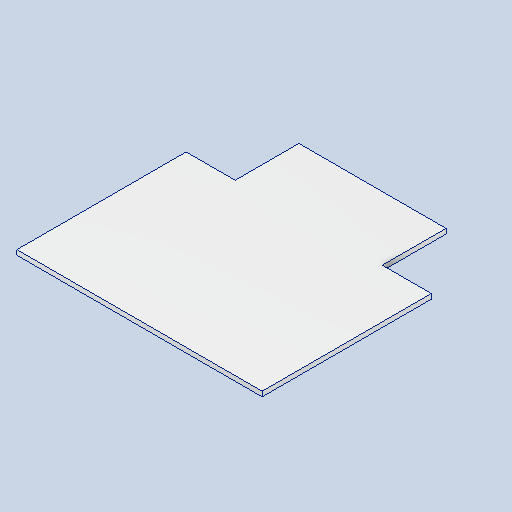
# Autodesk Inventor part: minisumopodsr
Saved by Autodesk Inventor 2022.3 (Build 263350000, 350)
## iProperties
Created: 2022-10-10
Part Number: minisumopodsr
Material: Aluminum 6061
Document SubType Name: Modeling
Designer: komputer
Density: 2.7 g/cm^3
Appearance: Aluminum - Flat
Author: komputer
Autodesk Inventor part; units mm, degrees
ref_plane "YZ Plane" through (0, 0, 0) normal (1, 0, 0) x (0, 1, 0)
ref_plane "XZ Plane" through (0, 0, 0) normal (0, 1, 0) x (-1, 0, 0)
ref_plane "XY Plane" through (0, 0, 0) normal (0, 0, 1) x (1, 0, 0)
sketch "Sketch1" plane through (0, 0, 0) normal (0, 1, 0) x (-1, 0, 0)
  line L0 (-95.7688, 101.9192) -> (4.2312, 101.9192)
  line L1 (4.2312, 101.9192) -> (4.2312, 1.9192)
  line L2 (4.2312, 1.9192) -> (-95.7688, 1.9192)
  line L3 (-95.7688, 1.9192) -> (-95.7688, 101.9192)
  line L4 (-95.7688, 1.9192) -> (4.2312, 1.9192)
  line L5 (4.2312, 1.9192) -> (4.2312, 6.9192)
  line L6 (4.2312, 6.9192) -> (-95.7688, 6.9192)
  line L7 (-95.7688, 6.9192) -> (-95.7688, 1.9192)
  line L8 (4.2312, 1.9192) -> (-15.7688, 1.9192)
  line L9 (-15.7688, 1.9192) -> (-15.7688, 32.9192)
  line L10 (-15.7688, 32.9192) -> (4.2312, 32.9192)
  line L11 (4.2312, 32.9192) -> (4.2312, 1.9192)
  line L12 (-95.7688, 1.9192) -> (-75.7688, 1.9192)
  line L13 (-75.7688, 1.9192) -> (-75.7688, 32.9192)
  line L14 (-75.7688, 32.9192) -> (-95.7688, 32.9192)
  line L15 (-95.7688, 32.9192) -> (-95.7688, 1.9192)
  point P0 (0, 0)
  dimension "d0" = 100
  dimension "d1" = 100
  dimension "d2" = 5
  dimension "d3" = 20
  dimension "d4" = 31
  dimension "d5" = 20
  constraints: 32 end point, 8 parallel, 4 horizontal, 4 perpendicular, 2 point on line
  measures "d0" distance of L1.end L2.end
  measures "d1" distance of L0.end L1.end
  measures "d2" distance of L5.end L4.end
  measures "d3" distance of L9.end L10.end
  measures "d4" distance of L8.end L9.end
  measures "d5" distance of L14.end L13.end
extrude "Extrusion1" add sketch "Sketch1" along normal blind 2 contours L0 L1 L10 L9 L6 L13 L14 L3 | L6 L9 L2 L13
sketch "Sketch2" plane through (0, 2, 0) normal (0, 1, 0) x (1, 0, 0)
  line L0 (-4.2312, -82.6348) -> (-4.2312, -11.6268) projected
  line L1 (95.7688, -11.6268) -> (95.7688, -82.6348) projected
  line L2 (75.7688, -32.9192) -> (75.7688, -1.9192) projected
  line L3 (15.7688, -1.9192) -> (15.7688, -32.9192) projected
  line L4 (75.7688, -1.9192) -> (15.7688, -1.9192)
  line L5 (15.7688, -1.9192) -> (15.7688, -6.9192)
  line L6 (15.7688, -6.9192) -> (75.7688, -6.9192)
  line L7 (75.7688, -6.9192) -> (75.7688, -1.9192)
  line L8 (95.7688, -82.6348) -> (-4.2312, -82.6348) projected
  line L9 (95.7688, -11.6268) -> (-4.2312, -11.6268) projected
  point P0 (0, 0)
  dimension "d8" = 5
  constraints: 8 end point, 2 parallel, 1 horizontal, 1 perpendicular, 1 point on line
  measures "d8" distance of L5.end L4.end
extrude "Extrusion2" cut sketch "Sketch2" against normal blind 2 contours L3 L4 L2 L6
body "Solid1"
